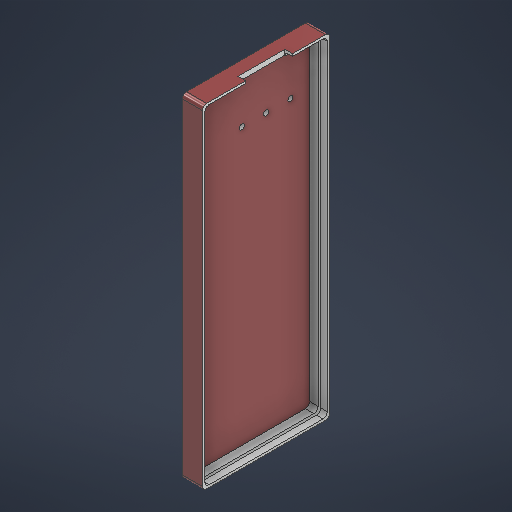
# Autodesk Inventor part: cDAQ_Lid_Box
Saved by Autodesk Inventor 2027 (Build 310192000, 192)
## iProperties
Created: 2026-05-08
Part Number: cDAQ_Lid_Box
Material: Generic
Document SubType Name: Modeling
Designer: giese
Density: 1 g/cm^3
Appearance: Default
Author: giese
Autodesk Inventor part; units mm, degrees
ref_plane "YZ Plane" through (0, 0, 0) normal (1, 0, 0) x (0, 1, 0)
ref_plane "XZ Plane" through (0, 0, 0) normal (0, 1, 0) x (-1, 0, 0)
ref_plane "XY Plane" through (0, 0, 0) normal (0, 0, 1) x (1, 0, 0)
sketch "Sketch1" plane through (0, 0, 0) normal (1, 0, 0) x (0, 1, 0)
  line L0 (50.7569, 48.4212) -> (-202.6081, 48.4212)
  line L1 (-202.6081, 48.4212) -> (-202.6081, -48.0988)
  line L2 (-202.6081, -48.0988) -> (50.7569, -48.0988)
  line L3 (50.7569, -48.0988) -> (50.7569, 48.4212)
  point P0 (0, 0)
  dimension "d0" = 96.52
  dimension "d1" = 253.365
  constraints: 8 end point, 2 parallel, 1 horizontal, 1 perpendicular
  measures "d0" distance of L2.end L0.start
  measures "d1" distance of L0.start L0.end
extrude "Extrusion1" add sketch "Sketch1" along normal blind 15.24
sketch "Sketch2" plane through (15.24, 0, 0) normal (1, 0, 0) x (0, 0, -1)
  line L0 (-44.6112, 46.9469) -> (44.2888, 46.9469)
  line L1 (44.2888, 46.9469) -> (44.2888, -198.7981)
  line L2 (44.2888, -198.7981) -> (-44.6112, -198.7981)
  line L3 (-44.6112, -198.7981) -> (-44.6112, 46.9469)
  line L4 (-48.4212, 50.7569) -> (-48.4212, -202.6081) projected
  line L5 (-48.4212, -202.6081) -> (48.0988, -202.6081) projected
  point P0 (0, 0)
  dimension "d4" = 88.9
  dimension "d5" = 245.745
  dimension "d6" = 3.81
  dimension "d7" = 3.81
  constraints: 8 end point, 2 parallel, 1 horizontal, 1 perpendicular
  measures "d4" distance of L0.start L0.end
  measures "d5" distance of L0.end L1.end
  measures "d6" distance between parallel lines of L4 L3
  measures "d7" distance between parallel lines of L5 L2
extrude "Extrusion2" cut sketch "Sketch2" against normal blind 11.43
sketch "Sketch3" plane through (0, 0, 0) normal (-1, 0, 0) x (0, 0, 1)
  circle A0 centre (-29.8108, 10.5233) radius 2
  line L0 (-48.0988, -202.6081) -> (-48.0988, 50.7569) projected
  line L1 (-48.0988, 50.7569) -> (48.4212, 50.7569) projected
  circle A1 centre (-11.312, 10.5233) radius 2
  circle A2 centre (7.1869, 10.5233) radius 2
  point P0 (0, 0)
  dimension "d10" = 18.288
  dimension "d11" = 40.2336
  dimension "d12" = 40.2336
  dimension "d13" = 18.4988
  dimension "d14" = 4
  dimension "d15" = 4
  dimension "d16" = 40.2336
  dimension "d17" = 18.4988
  dimension "d18" = 36.9976
  dimension "d21" = 4
  constraints: 3 centre point
  measures "d10" distance from line of L0 A0.centre
  measures "d11" distance from line of L1 A0.centre
  measures "d12" distance from line of L1 A1.centre
  measures "d13" distance of A0.centre A1.centre
  measures "d14" diameter of A1
  measures "d15" diameter of A2
  measures "d16" distance from line of L1 A2.centre
  measures "d17" distance of A1.centre A2.centre
  measures "d18" distance of A0.centre A2.centre
  measures "d21" diameter of A0
extrude "Extrusion3" cut sketch "Sketch3" against normal blind 3.81
sketch "Sketch6" plane through (0, 50.7569, 48.4212) normal (0, 1, 0) x (1, 0, 0)
  line L0 (15.24, 3.81) -> (15.24, 92.71) projected
  line L1 (9.4234, 32.7559) -> (15.24, 32.7559)
  line L2 (15.24, 32.7559) -> (15.24, 68.326)
  line L3 (15.24, 68.326) -> (9.4234, 68.326)
  line L4 (9.4234, 68.326) -> (9.4234, 32.7559)
  line L5 (0, 96.52) -> (15.24, 96.52) projected
  point P0 (0, 48.4212)
  point P1 (12.3317, 68.326)
  point P2 (12.3317, 32.7559)
  dimension "d30" = 5.8166
  dimension "d31" = 35.5701
  dimension "d32" = 28.194
  constraints: 8 end point, 2 midpoint, 2 parallel, 1 horizontal, 1 perpendicular, 1 point on line
  measures "d30" distance between parallel lines of L0 L4
  measures "d31" distance of point (12.332, 68.326) point (12.332, 32.756)
  measures "d32" distance between parallel lines of L5 L3
extrude "Extrusion5" cut sketch "Sketch6" against normal blind 3.81
fillet "Fillet1" radius 3.175 4 edges at (7.62, 50.7569, -48.0988) (7.62, 50.7569, 48.4212) (7.62, -202.6081, 48.4212) (7.62, -202.6081, -48.0988)
sketch "Sketch7" plane through (15.24, 0, 0) normal (1, 0, 0) x (0, 0, -1)
  line L0 (-44.6112, -198.7981) -> (-44.6112, 46.9469) projected
  line L1 (-44.6112, 46.9469) -> (-42.3252, 46.9469)
  line L2 (-42.3252, 48.9469) -> (-46.6112, 48.9469)
  line L3 (-46.6112, 48.9469) -> (-46.6112, 48.4709)
  line L4 (-44.6112, -192.7021) -> (-44.6112, -198.7981)
  line L5 (44.2888, -198.7981) -> (-44.6112, -198.7981) projected
  line L6 (-42.3252, -200.7981) -> (-46.6112, -200.7981)
  line L7 (-46.6112, -200.7981) -> (-46.6112, -192.7021)
  line L8 (44.2888, 46.9469) -> (44.2888, -198.7981) projected
  line L9 (44.2888, -192.7021) -> (44.2888, -198.7981)
  line L10 (44.2888, -198.7981) -> (42.0028, -198.7981)
  line L11 (44.2888, -198.7981) -> (44.2888, -192.7021)
  line L12 (46.2888, -192.7021) -> (46.2888, -200.7981)
  line L13 (46.2888, -200.7981) -> (42.0028, -200.7981)
  line L14 (-44.6112, 46.9469) -> (44.2888, 46.9469) projected
  line L15 (42.0028, 46.9469) -> (44.2888, 46.9469)
  line L16 (46.2888, 48.4709) -> (46.2888, 48.9469)
  line L17 (46.2888, 48.9469) -> (42.0028, 48.9469)
  line L18 (-42.3252, 48.9469) -> (42.0028, 48.9469)
  line L19 (42.0028, 46.9469) -> (-42.3252, 46.9469)
  line L20 (46.2888, 48.4709) -> (46.2888, -192.7021)
  line L21 (44.2888, -192.7021) -> (44.2888, 46.9469)
  line L22 (42.0028, -198.7981) -> (-42.3252, -198.7981)
  line L23 (-42.3252, -200.7981) -> (42.0028, -200.7981)
  line L24 (-46.6112, -192.7021) -> (-46.6112, 48.4709)
  line L25 (-44.6112, 46.9469) -> (-44.6112, -192.7021)
  point P0 (0, 0)
  point P1 (-44.6112, 48.4709)
  point P2 (-44.2302, 48.9789)
  point P3 (44.2888, 48.4709)
  dimension "d34" = 2
  dimension "d35" = 2
  dimension "d38" = 2
  dimension "d39" = 2
  dimension "d42" = 2
  dimension "d43" = 2
  dimension "d46" = 2
  dimension "d47" = 2
  constraints: 44 end point, 9 point on line, 4 parallel, 4 perpendicular, 2 collinear, 2 horizontal, 2 vertical
  measures "d34" distance between parallel lines of L2 L1
  measures "d35" distance between parallel lines of L0 L3
  measures "d38" distance between parallel lines of L7 L0
  measures "d39" distance between parallel lines of L5 L6
  measures "d42" distance between parallel lines of L5 L13
  measures "d43" distance between parallel lines of L8 L12
  measures "d46" distance between parallel lines of L14 L17
  measures "d47" distance between parallel lines of L8 L16
extrude "Extrusion6" cut sketch "Sketch7" against normal blind 5
fillet "Fillet2" radius 3.175 8 edges at (12.74, 48.9469, 46.6112) (7.025, 46.9469, 44.6112) (12.74, 48.9469, -46.2888) (7.025, 46.9469, -44.2888) (7.025, -198.7981, 44.6112) (12.74, -200.7981, 46.6112) (7.025, -198.7981, -44.2888) (12.74, -200.7981, -46.2888)
body "Solid1"
